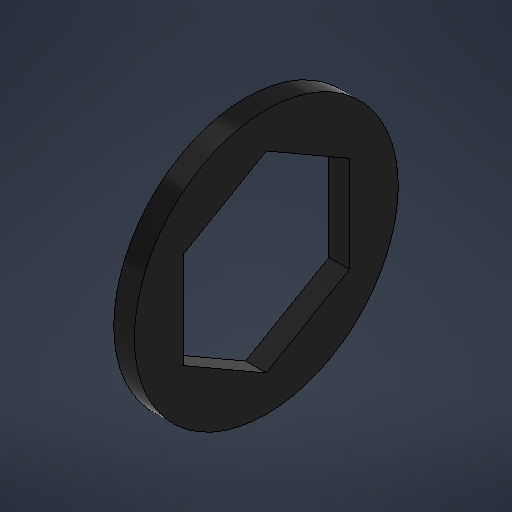
# Autodesk Inventor part: 3DPRINT,REVERSERGEAR,SPACER,SHORT
Saved by Autodesk Inventor 2026.1 (Build 301233020, 233B)
## iProperties
Created: 2026-02-15
Part Number: 3DPRINT,REVERSERGEAR,SPACER,SHORT
Material: ABS Plastic
Document SubType Name: Modeling
Designer: Owen L
Density: 1.06 g/cm^3
Appearance: Smooth - Black
Author: Owen L
Autodesk Inventor part; units mm, degrees
ref_plane "YZ Plane" through (0, 0, 0) normal (1, 0, 0) x (0, 1, 0)
ref_plane "XZ Plane" through (0, 0, 0) normal (0, 1, 0) x (-1, 0, 0)
ref_plane "XY Plane" through (0, 0, 0) normal (0, 0, 1) x (1, 0, 0)
sketch "Sketch1" plane through (0, 0, 0) normal (1, 0, 0) x (0, 1, 0)
  line L0 (-3.7028, 6.4135) -> (3.7028, 6.4135)
  line L1 (3.7028, 6.4135) -> (7.4057, 0)
  line L2 (7.4057, 0) -> (3.7028, -6.4135)
  line L3 (3.7028, -6.4135) -> (-3.7028, -6.4135)
  line L4 (-3.7028, -6.4135) -> (-7.4057, 0)
  line L5 (-7.4057, 0) -> (-3.7028, 6.4135)
  circle A0 centre (0, 0) radius 10.16
  dimension "d0" = 12.827
  dimension "d1" = 20.32
  constraints: 12 end point, 2 coincident, 1 centre point, 1 horizontal, 13 other
  measures "d0" distance between parallel lines of L3 L0
  measures "d1" diameter of A0
extrude "Extrusion1" add sketch "Sketch1" along normal blind 1.5875
body "Solid1"
